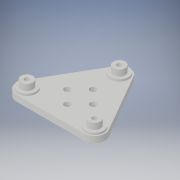
# Autodesk Inventor part: PlanetaryHolderTop
Saved by Autodesk Inventor 2018.3 (Build 223284000, 284)
## iProperties
Created: 2018-07-08
Part Number: PlanetaryHolderTop
Material: Generisch
Document SubType Name: Modeling
Designer: JochenAlt
Density: 1 g/cm^3
Appearance: Vorgabe
Author: JochenAlt
Autodesk Inventor part; units mm, degrees
ref_plane "YZ Plane" through (0, 0, 0) normal (1, 0, 0) x (0, 1, 0)
ref_plane "XZ Plane" through (0, 0, 0) normal (0, 1, 0) x (-1, 0, 0)
ref_plane "XY Plane" through (0, 0, 0) normal (0, 0, 1) x (1, 0, 0)
sketch "Skizze1" plane through (0, 0, 0) normal (0, 0, 1) x (1, 0, 0)
  circle A0 centre (0, 0) radius 19.21 construction
  circle A1 centre (0, 0) radius 9.75
  circle A2 centre (0, 19.21) radius 1.15
  line L0 (0, 0) -> (-16.6363, -9.605) construction
  line L1 (0, 33.791) -> (0, -28.0435) construction
  line L2 (-32.657, 0) -> (32.657, 0) construction
  circle A3 centre (0, 0) radius 6.35 construction
  circle A4 centre (0, 6.35) radius 1.5
  circle A5 centre (0, -6.35) radius 1.5
  circle A6 centre (6.35, 0) radius 1.5
  circle A7 centre (-6.35, 0) radius 1.5
  arc A8 (0, 24.36) -> (-4.46, 21.785) centre (0, 19.21) ccw
  circle A9 centre (16.6363, -9.605) radius 1.15
  arc A10 (16.6363, -14.755) -> (21.0964, -7.03) centre (16.6363, -9.605) ccw
  circle A11 centre (-16.6363, -9.605) radius 1.15
  arc A12 (-21.0964, -7.03) -> (-16.6363, -14.755) centre (-16.6363, -9.605) ccw
  circle A13 centre (0, 19.21) radius 2.9
  circle A14 centre (16.6363, -9.605) radius 2.9
  circle A15 centre (-16.6363, -9.605) radius 2.9
  circle A16 centre (0, 19.21) radius 4.5
  circle A17 centre (16.6363, -9.605) radius 4.5
  circle A18 centre (-16.6363, -9.605) radius 4.5
  line L3 (-4.46, 21.785) -> (-21.0964, -7.03)
  line L4 (-16.6363, -14.755) -> (16.6363, -14.755)
  line L5 (4.46, 21.785) -> (21.0964, -7.03)
  arc A19 (4.46, 21.785) -> (0, 24.36) centre (0, 19.21) ccw
  circle A20 centre (0, 19.21) radius 2.1 construction
  line L6 (1.2124, 21.31) -> (2.4249, 19.21)
  line L7 (2.4249, 19.21) -> (1.2124, 17.11)
  line L8 (1.2124, 17.11) -> (-1.2124, 17.11)
  line L9 (-1.2124, 17.11) -> (-2.4249, 19.21)
  line L10 (-2.4249, 19.21) -> (-1.2124, 21.31)
  line L11 (-1.2124, 21.31) -> (1.2124, 21.31)
  circle A21 centre (-16.6363, -9.605) radius 2.1 construction
  circle A22 centre (16.6363, -9.605) radius 2.1 construction
  line L12 (-17.8473, -11.7058) -> (-19.0612, -9.6067)
  line L13 (-19.0612, -9.6067) -> (-17.8502, -7.5058)
  line L14 (-17.8502, -7.5058) -> (-15.4254, -7.5042)
  line L15 (-15.4254, -7.5042) -> (-14.2115, -9.6033)
  line L16 (-14.2115, -9.6033) -> (-15.4225, -11.7042)
  line L17 (-15.4225, -11.7042) -> (-17.8473, -11.7058)
  line L18 (15.7481, -11.8613) -> (14.2382, -9.9639)
  line L19 (14.2382, -9.9639) -> (15.1264, -7.7076)
  line L20 (15.1264, -7.7076) -> (17.5246, -7.3487)
  line L21 (17.5246, -7.3487) -> (19.0345, -9.2461)
  line L22 (19.0345, -9.2461) -> (18.1462, -11.5024)
  line L23 (18.1462, -11.5024) -> (15.7481, -11.8613)
  point P0 (0, 21.31)
  point P1 (-16.6363, -9.605)
  point P2 (-16.6349, -11.705)
  point P3 (16.9472, -11.6819)
  dimension "d31" = 4.2
  dimension "d0" = 38.42
  dimension "d1" = 2.3
  dimension "d2" = 30
  dimension "d3" = 19.5
  dimension "d4" = 12.7
  dimension "d5" = 3
  dimension "d8" = 4
  dimension "d26" = 5.8
  dimension "d30" = 9
  constraints: 44 end point, 20 centre point, 19 coincident, 16 point on circle, 12 equal radius, 7 point on line, 6 tangent, 3 midpoint, 1 concentric, 1 symmetric about line, 1 vertical alignment, 48 other
  measures "d0" diameter of A0
  measures "d1" diameter of A2
  measures "d2" angle of L0 L2
  measures "d3" diameter of A1
  measures "d4" diameter of A3
  measures "d5" diameter of A4
  measures "d8" radial gap between concentric circles of A2 A8
  measures "d26" diameter of A13
  measures "d30" diameter of A16
extrude "Extrusion1" add sketch "Skizze1" along normal blind 3 contours A1 | A19 L5 A10 L4 A12 L3 A8 | A13 | A14 | A15 | A16 | A17 | A18 | L6 L7 L8 L9 L10 L11 | L12 L13 L14 L15 L16 L17 | L18 L19 L20 L21 L22 L23
extrude "Extrusion3" cut sketch "Skizze1" along normal blind 1.5 contours A1
extrude "Extrusion4" add sketch "Skizze1" along normal blind 1 from surface at 3 contours A13 | A14 | A15 | A16 | A17 | A18 | L6 L7 L8 L9 L10 L11 | L12 L13 L14 L15 L16 L17 | L18 L19 L20 L21 L22 L23
extrude "Extrusion6" add sketch "Skizze1" along normal blind 3 from surface at 4 contours A13 | A14 | A15 | L6 L7 L8 L9 L10 L11 | L12 L13 L14 L15 L16 L17 | L18 L19 L20 L21 L22 L23
extrude "Extrusion8" cut sketch "Skizze1" along normal blind 1.5 contours L6 L7 L8 L9 L10 L11 | L12 L13 L14 L15 L16 L17 | L18 L19 L20 L21 L22 L23
